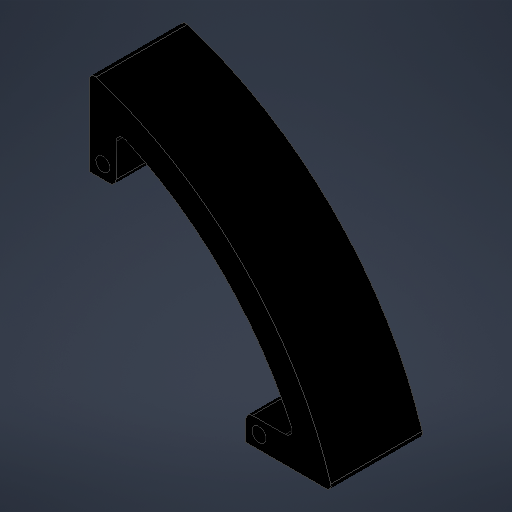
# Autodesk Inventor part: Side Wall
Saved by Autodesk Inventor 2026.1 (Build 301233020, 233B)
## iProperties
Created: 2025-11-06
Part Number: Side Wall
Material: Generic
Document SubType Name: Modeling
Designer: Bahaa
Density: 1 g/cm^3
Appearance: Default
Author: Bahaa
Autodesk Inventor part; units mm, degrees
ref_plane "YZ Plane" through (0, 0, 0) normal (1, 0, 0) x (0, 1, 0)
ref_plane "XZ Plane" through (0, 0, 0) normal (0, 1, 0) x (-1, 0, 0)
ref_plane "XY Plane" through (0, 0, 0) normal (0, 0, 1) x (1, 0, 0)
sketch "Sketch1" plane through (0, 0, 0) normal (0, 1, 0) x (-1, 0, 0)
  line L0 (-130, 30) -> (130, 30)
  line L1 (130, 30) -> (130, -30)
  line L2 (130, -30) -> (-130, -30)
  line L3 (-130, -30) -> (-130, 30)
  line L4 (-130, 30) -> (130, -30) construction
  line L5 (130, 30) -> (-130, -30) construction
  line L6 (-30, -130) -> (-30, 130)
  line L7 (-30, 130) -> (30, 130)
  line L8 (30, 130) -> (30, -130)
  line L9 (30, -130) -> (-30, -130)
  line L10 (-30, -130) -> (30, 130) construction
  line L11 (-30, 130) -> (30, -130) construction
  line L12 (130, -30) -> (-130, -30)
  line L13 (-130, -30) -> (-130, 30)
  line L14 (-130, 30) -> (130, 30)
  line L15 (130, 30) -> (130, -30)
  line L16 (130, -30) -> (-130, 30) construction
  line L17 (-130, -30) -> (130, 30) construction
  line L18 (30, 130) -> (30, -130)
  line L19 (30, -130) -> (-30, -130)
  line L20 (-30, -130) -> (-30, 130)
  line L21 (-30, 130) -> (30, 130)
  line L22 (30, 130) -> (-30, -130) construction
  line L23 (30, -130) -> (-30, 130) construction
  arc A0 (130, -30) -> (130, 30) centre (0, 0) ccw
  line L24 (-130, 0) -> (-107.5, 0) construction
  circle A1 centre (0, 0) radius 107.5
  circle A2 centre (0, 0) radius 92.5
  line L25 (-30, 87.5) -> (-30, 77)
  line L26 (-30, 77) -> (-38, 77)
  circle A3 centre (0, 0) radius 99.5
  line L27 (-38, 77) -> (-38, 91.9579)
  line L28 (-87.5, 30) -> (-77, 30)
  line L29 (-77, 30) -> (-77, 38)
  line L30 (-77, 38) -> (-91.9579, 38)
  line L31 (-34, 77) -> (-34, 81) construction
  line L32 (-77, 34) -> (-81, 34) construction
  line L33 (-81, 34) -> (-81, 30) construction
  point P0 (-30, 30)
  point P1 (-30, 30)
  point P2 (-30, 77)
  point P3 (-30, 103.2291)
  point P4 (-103.2291, 30)
  point P5 (-77, 30)
  dimension "d1" = 260
  dimension "d2" = 60
  dimension "d5" = 360
  dimension "d7" = 22.5
  dimension "d8" = 15
  dimension "d9" = 10.5
  dimension "d10" = 8
  dimension "d11" = 8
  dimension "d12" = 10.5
  dimension "d13" = 8
  dimension "d14" = 4
  dimension "d15" = 4
  dimension "d16" = 4
  constraints: 68 end point, 7 coincident, 7 point on line, 6 point on circle, 5 midpoint, 4 perpendicular, 3 centre point, 3 horizontal, 2 parallel, 2 vertical, 46 other
  measures "d1" distance of L1.end L2.end
  measures "d2" distance of L0.end L1.end
  measures "d7" distance of L24.start L24.end
  measures "d9" distance of L25.start L25.end
  measures "d10" distance of L25.end L26.end
  measures "d12" distance of L28.start L28.end
  measures "d13" distance of L28.end L29.end
  measures "d14" distance of L31.start L31.end
  measures "d15" distance of L32.start L32.end
  measures "d16" distance of L32.end L33.end
extrude "Extrusion1" add sketch "Sketch1" along normal blind 27.5 contours A2 L30 L29 L0 | L0 A3 L30 A2 | L0 A1 L6 A3 | L27 A3 L6 A2 | A2 L6 L26 L27
fillet "Fillet1" radius 2 4 edges at (38, 13.75, 91.9579) (91.9579, 13.75, 38) (77, 13.75, 38) (38, 13.75, 77)
hole "Hole1" at (34, 0, 81) at (81, 0, 34) direction (0, 1, 0) diameter 4.2 depth 6
ref_plane "Work Plane1" through (0, 13.75, 0) normal (0, 1, 0) x (1, 0, 0)
mirror "Mirror1" about plane through (0, 13.75, 0) normal (0, 1, 0) of "Hole1"
fillet "Fillet2" radius 1.5 2 edges at (103.2291, 13.75, 30) (30, 13.75, 103.2291)
equation "\"d9\" = d12"
equation "\"d10\" = d11"
equation "\"d13\" = d11"
equation "\"d14\" = 0.5 * d11"
equation "\"d15\" = 0.5 * d11"
equation "\"d16\" = 0.5 * d11"
body "Solid1"
